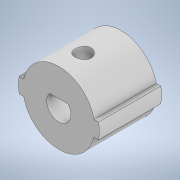
# Autodesk Inventor part: Переходник с дифференциала на ось 3мм
Saved by Autodesk Inventor 2020 (Build 240168000, 168)
## iProperties
Created: 2021-05-24
Part Number: Переходник с дифференциала на ось 3мм
Material: Типовые
Document SubType Name: Обычные детали
Designer: Антон
Density: 1 g/cm^3
Appearance: По умолчанию
Author: Антон
Autodesk Inventor part; units mm, degrees
ref_plane "YZ Plane" through (0, 0, 0) normal (1, 0, 0) x (0, 1, 0)
ref_plane "XZ Plane" through (0, 0, 0) normal (0, 1, 0) x (-1, 0, 0)
ref_plane "XY Plane" through (0, 0, 0) normal (0, 0, 1) x (1, 0, 0)
sketch "Эскиз1" plane through (0, 0, 0) normal (0, 0, 1) x (1, 0, 0)
  circle A0 centre (0, 0) radius 4.45
  line L0 (-5, 0.95) -> (5, 0.95)
  line L1 (5, 0.95) -> (5, -0.95)
  line L2 (5, -0.95) -> (-5, -0.95)
  line L3 (-5, -0.95) -> (-5, 0.95)
  line L4 (-5, 0.95) -> (5, -0.95) construction
  line L5 (5, 0.95) -> (-5, -0.95) construction
  circle A1 centre (0, 0) radius 5
  point P0 (-4.3474, -0.95)
  point P1 (4.3474, -0.95)
  point P2 (4.3474, 0.95)
  point P3 (-4.3474, 0.95)
  point P4 (4.9089, -0.95)
  point P5 (4.9089, 0.95)
  point P6 (-4.9089, 0.95)
  point P7 (-4.9089, -0.95)
  dimension "d0" = 8.9
  dimension "d1" = 1.9
  dimension "d5" = 10
  constraints: 12 end point, 2 centre point, 2 coincident, 2 midpoint, 2 parallel, 1 horizontal, 1 perpendicular, 1 tangent
  measures "d0" diameter of A0
  measures "d1" distance of L0.end L1.end
  measures "d5" diameter of A1
extrude "Выдавливание1" add sketch "Эскиз1" along normal blind 7.7 contours A0 L2 L0 | A0 L0 A1 L2 | L0 A0 | A0 L2 | A0 L2 A1 L0
sketch "Эскиз2" plane through (0, 0, 7.7) normal (0, 0, 1) x (1, 0, 0)
  circle A0 centre (0, 0) radius 1.5
  line L0 (-1.5, 1) -> (1.5, 1)
  line L1 (1.5, 1) -> (1.5, -1)
  line L2 (1.5, -1) -> (-1.5, -1)
  line L3 (-1.5, -1) -> (-1.5, 1)
  line L4 (-1.5, 1) -> (1.5, -1) construction
  line L5 (1.5, 1) -> (-1.5, -1) construction
  point P0 (1.118, 1)
  point P1 (-1.118, 1)
  dimension "d6" = 3
  dimension "d8" = 2
  constraints: 12 end point, 2 midpoint, 2 parallel, 1 centre point, 1 coincident, 1 horizontal, 1 perpendicular, 1 tangent
  measures "d6" diameter of A0
  measures "d8" distance of L0.end L1.end
extrude "Выдавливание2" cut sketch "Эскиз2" against normal blind 5 contours A0 L2 L0 | A0 L2
sketch "Эскиз3" plane through (-1.118, 1, 7.7) normal (0, -1, 0) x (1, 0, 0)
  line L0 (0, -5) -> (2.2361, -5) projected
  line L1 (1.118, -5) -> (1.118, 0)
  line L2 (0, 0) -> (2.2361, 0) projected
  circle A0 centre (1.118, -3) radius 1
  point P0 (1.118, -7.7)
  dimension "d11" = 2
  dimension "d13" = 2
  constraints: 2 end point, 2 midpoint, 1 centre point, 1 point on line
  measures "d11" diameter of A0
  measures "d13" distance from line of L0 A0.centre
extrude "Выдавливание3" cut sketch "Эскиз3" along normal through all both and the other way through all
equation "\"Радиус_гибки\" = Толщина"
equation "\"Ширина_просечки\" = Толщина"
equation "\"Глубина_просечки\" = 0.5 * Толщина"
equation "\"Размер_просечки\" = 4 * Толщина"
equation "\"Мин_остаток\" = 2 * Толщина"
equation "\"Радиус_перехода\" = Радиус_гибки"
equation "\"Радиус_Якоби\" = Толщина"
equation "\"Размер_зазора\" = Толщина"
equation "\"Толщина\" = 0.5"
